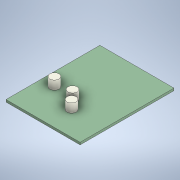
# Autodesk Inventor part: MotorDriverShield
Saved by Autodesk Inventor 2022.2 (Build 262287010, 287A)
## iProperties
Created: 2022-03-26
Part Number: MotorDriverShield
Material: Generic
Document SubType Name: Modeling
Designer: Santiago Larraín
Density: 1 g/cm^3
Appearance: Default
Author: Santiago Larraín
Autodesk Inventor part; units mm, degrees
ref_plane "YZ Plane" through (0, 0, 0) normal (1, 0, 0) x (0, 1, 0)
ref_plane "XZ Plane" through (0, 0, 0) normal (0, 1, 0) x (-1, 0, 0)
ref_plane "XY Plane" through (0, 0, 0) normal (0, 0, 1) x (1, 0, 0)
sketch "Sketch1" plane through (0, 0, 0) normal (0, 1, 0) x (-1, 0, 0)
  line L0 (0, 0) -> (0, -65)
  line L1 (0, -65) -> (51.3, -65)
  line L2 (51.3, -65) -> (51.3, 0)
  line L3 (51.3, 0) -> (0, 0)
  dimension "d0" = 65
  dimension "d1" = 51.3
  constraints: 8 end point, 2 parallel, 1 perpendicular, 1 vertical
  measures "d0" distance of L0.start L0.end
  measures "d1" distance of L1.end L0.end
extrude "Extrusion1" add sketch "Sketch1" along normal blind 1.575
sketch "Sketch2" plane through (0, 1.575, 0) normal (0, 1, 0) x (1, 0, 0)
  line L0 (-51.3, 65) -> (-51.3, 0) projected
  line L1 (-51.3, 0) -> (-51.3, 24.5)
  line L2 (-51.3, 24.5) -> (-42.3, 24.5)
  line L3 (-42.3, 24.5) -> (-42.3, 0)
  line L4 (-42.3, 0) -> (-51.3, 0)
  circle A0 centre (-42.3, 24.5) radius 3.15
  line L5 (-51.3, 0) -> (-51.3, 23)
  line L6 (-51.3, 23) -> (-28.2, 23)
  line L7 (-28.2, 23) -> (-28.2, 0)
  line L8 (-28.2, 0) -> (-51.3, 0)
  circle A1 centre (-28.2, 23) radius 3.15
  line L9 (-51.3, 0) -> (-51.3, 28.7)
  line L10 (-51.3, 28.7) -> (-34.6, 28.7)
  line L11 (-34.6, 28.7) -> (-34.6, 0)
  line L12 (-34.6, 0) -> (-51.3, 0)
  line L13 (-51.3, 0) -> (-51.3, 16.7)
  line L14 (-51.3, 16.7) -> (-22.6, 16.7)
  line L15 (-22.6, 16.7) -> (-22.6, 0)
  line L16 (-22.6, 0) -> (-51.3, 0)
  circle A2 centre (-22.6, 16.7) radius 3.15
  point P0 (0, 0)
  dimension "d4" = 24.5
  dimension "d5" = 9
  dimension "d6" = 6.3
  dimension "d7" = 23
  dimension "d8" = 23.1
  dimension "d9" = 6.3
  dimension "d10" = 28.7
  dimension "d11" = 16.7
  dimension "d12" = 16.7
  dimension "d13" = 28.7
  dimension "d14" = 6.3
  constraints: 32 end point, 8 parallel, 4 perpendicular, 4 point on line, 3 centre point, 3 coincident
  measures "d4" distance of L0.end L1.end
  measures "d5" distance of L1.end L2.end
  measures "d6" diameter of A0
  measures "d7" distance of L0.end L5.end
  measures "d8" distance of L5.end L6.end
  measures "d9" diameter of A1
  measures "d10" distance of L0.end L9.end
  measures "d11" distance of L9.end L10.end
  measures "d12" distance of L0.end L13.end
  measures "d13" distance of L13.end L14.end
  measures "d14" diameter of A2
extrude "Extrusion2" add sketch "Sketch2" along normal blind 6.1 contours A0 L6 L3 L2 | L2 L3 L6 A0 | L6 L3 A0 | A0 L3 L6 | A1 L7 L6 | L6 L7 A1 | A2 L15 L14 | L14 L15 A2
body "Solid1"
